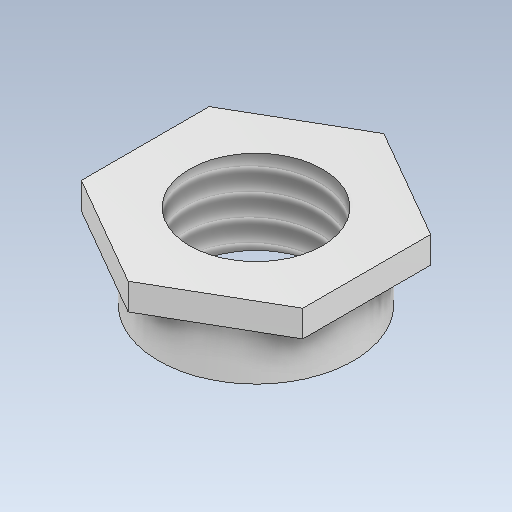
# Autodesk Inventor part: SF319
Saved by Autodesk Inventor 2020.4 (Build 244396000, 396)
## iProperties
Created: 2021-09-10
Part Number: SF319
Material: 鉄、ダクタイル鋳鉄
Document SubType Name: Modeling
Designer: naoki
Density: 7.15 g/cm^3
Appearance: サテン
Description: 既製品
Mass: 0.138188 g
Surface Area: 0.754334 cm^2
Volume: 0.019327 cm^3
Author: Naoki Iwasawa
Comments: https://jp.misumi-ec.com/vona2/detail/221000555673/?HissuCode=SF319
Autodesk Inventor part; units mm, degrees
ref_plane "YZ Plane" through (0, 0, 0) normal (1, 0, 0) x (0, 1, 0)
ref_plane "XZ Plane" through (0, 0, 0) normal (0, 1, 0) x (-1, 0, 0)
ref_plane "XY Plane" through (0, 0, 0) normal (0, 0, 1) x (1, 0, 0)
sketch "スケッチ1" plane through (0, 0, 0) normal (0, 1, 0) x (-1, 0, 0)
  circle A0 centre (0, 0) radius 1.5
  circle A1 centre (0, 0) radius 2.2
  circle A2 centre (0, 0) radius 2.5 construction
  line L0 (2.5, 1.4434) -> (2.5, -1.4434)
  line L1 (2.5, -1.4434) -> (0, -2.8868)
  line L2 (0, -2.8868) -> (-2.5, -1.4434)
  line L3 (-2.5, -1.4434) -> (-2.5, 1.4434)
  line L4 (-2.5, 1.4434) -> (0, 2.8868)
  line L5 (0, 2.8868) -> (2.5, 1.4434)
  line L6 (0, 4.5564) -> (0, -4.4801) construction
  line L7 (3.3581, 0) -> (-3.3581, 0) construction
  point P0 (1.25, 2.1651)
  dimension "d2" = 5
  dimension "d0" = 4.4
  dimension "d1" = 3
  constraints: 16 end point, 4 coincident, 3 midpoint, 3 point on line, 2 centre point, 1 horizontal, 1 vertical, 16 other
  measures "d0" diameter of A1
  measures "d1" diameter of A0
extrude "押し出し1" add sketch "スケッチ1" along normal blind 0.6 contours A1 | L0 L1 L2 L3 L4 L5
extrude "押し出し2" add sketch "スケッチ1" against normal blind 1.3 contours A1
thread "ねじ1" size "M3x0.5" class "6H" standard "ANSI Metric M Profile" full length
